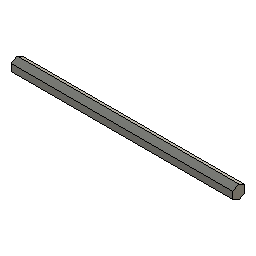
External1 (Autodesk Fusion 360 design; units mm, degrees)
part number: 2026-05-19-16-10-02-554
Autodesk Fusion 360 part; units mm, degrees
sketch "Sketch1" plane through (0, 0, 0) normal (1, 0, 0) x (0, 1, 0)
  line L0 (150, 45.3) -> (154.0703, 47.65)
  line L1 (154.0703, 47.65) -> (154.0703, 52.35)
  line L2 (154.0703, 52.35) -> (150, 54.7)
  line L3 (150, 54.7) -> (145.9297, 52.35)
  line L4 (145.9297, 52.35) -> (145.9297, 47.65)
  line L5 (145.9297, 47.65) -> (150, 45.3)
  point P0 (150, 50)
  dimension "d1" = 4.7
  measures "d1" distance of L0.start P0
extrude "Extrude1" add sketch "Sketch1" against normal blind 150
